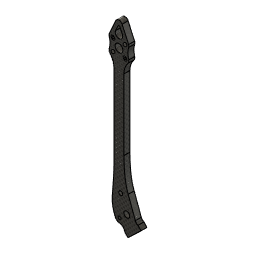
frame_assy_lab_9 (Autodesk Fusion 360 archive; units mm, degrees)
design "arm_rear_6mm"
Autodesk Fusion 360 part; units mm, degrees
(part 1 of 5)
sketch "Sketch1" plane through (0, 0, 0) normal (0, 0, 1) x (1, 0, 0)
  circle A0 centre (0, 0) radius 3.95
  line L0 (0, 0) -> (0, -178.3291)
  line L1 (-5, 0) -> (-5, -178.3291)
  line L2 (5, 0) -> (5, -178.3291)
  dimension "d1" = 7.9
  dimension "d2" = 5
  dimension "d3" = -5
  constraint coincident A0.centre L0.start
  constraint vertical L0
  measures "d1" diameter of A0
sketch "Sketch2" plane through (0, 0, 0) normal (0, 0, 1) x (1, 0, 0)
  circle A0 centre (0, 0) radius 3.95
  line L0 (0, 0) -> (-9, 0) construction
  line L1 (7.566, -7.566) -> (4.5962, -4.5962) construction
  line L2 (6.7175, 4.5962) -> (7.566, 5.4447)
  line L3 (4.5962, -6.7175) -> (5.4447, -7.566)
  line L4 (0.9091, 19.0167) -> (3.409, 13.5625)
  circle A1 centre (6.5054, -6.5054) radius 3.5
  line L5 (-4.5962, 6.7175) -> (-5.4447, 7.566)
  arc A2 (4.5962, 6.7175) -> (6.7175, 4.5962) centre (5.6569, 5.6569) ccw
  arc A3 (-7.566, -5.4447) -> (-5.4447, -7.566) centre (-6.5054, -6.5054) ccw
  arc A4 (9.1588, -8.7878) -> (5, -20) centre (22.1936, -20) ccw
  line L6 (7.566, -5.4447) -> (6.7175, -4.5962)
  arc A5 (9.8421, 5.4488) -> (9.8421, -5.4488) centre (27.0494, 0) ccw
  arc A6 (-4.5962, -6.7175) -> (-6.7175, -4.5962) centre (-5.6569, -5.6569) ccw
  circle A7 centre (0, 21) radius 3.5
  circle A8 centre (0, 12) radius 3.75
  line L7 (-5, -20) -> (5, -20) construction
  line L8 (-0.9091, 19.0167) -> (-3.409, 13.5625)
  arc A9 (5.4447, -7.566) -> (7.566, -5.4447) centre (6.5054, -6.5054) ccw
  line L9 (-6.7175, -4.5962) -> (-7.566, -5.4447)
  arc A10 (-5, -20) -> (-9.1588, -8.7878) centre (-22.1936, -20) ccw
  line L10 (5.4447, 7.566) -> (4.5962, 6.7175)
  line L11 (0, 0) -> (18.7579, 0) construction
  circle A11 centre (-6.5054, -6.5054) radius 3.5
  line L12 (-9.6985, 7.9385) -> (-3.1931, 22.4331)
  arc A12 (6.7175, -4.5962) -> (4.5962, -6.7175) centre (5.6569, -5.6569) ccw
  arc A13 (7.566, 5.4447) -> (5.4447, 7.566) centre (6.5054, 6.5054) ccw
  circle A14 centre (-6.5054, 6.5054) radius 3.5
  line L13 (0, 0) -> (13.2638, -13.2638) construction
  line L14 (0, 24.5) -> (0, 0) construction
  line L15 (9.6985, 7.9385) -> (3.1931, 22.4331)
  arc A15 (-6.7175, 4.5962) -> (-4.5962, 6.7175) centre (-5.6569, 5.6569) ccw
  line L16 (-5.4447, -7.566) -> (-4.5962, -6.7175)
  line L17 (-7.566, 5.4447) -> (-6.7175, 4.5962)
  arc A16 (-5.4447, 7.566) -> (-7.566, 5.4447) centre (-6.5054, 6.5054) ccw
  arc A17 (-9.8421, -5.4488) -> (-9.8421, 5.4488) centre (-27.0494, 0) ccw
  circle A18 centre (6.5054, 6.5054) radius 3.5
  arc A19 (0.9091, 19.0167) -> (-0.9091, 19.0167) centre (0, 18.6) ccw
  arc A20 (16.4975, -142.4127) -> (19.1132, -145.1691) centre (20.2426, -141.4781) ccw
  circle A21 centre (28.5466, -163.0999) radius 2.95 construction
  line L18 (36.8072, -178.2122) -> (44.0178, -178.0032) construction
  line L19 (-6.1772, -125.1087) -> (-6.7634, -132.2985)
  line L20 (0.7848, -157.6755) -> (0.9047, -157.0861) construction
  arc A22 (12.4548, -169.2574) -> (12.1429, -164.1911) centre (12.0783, -166.7378) ccw construction
  circle A23 centre (0.6152, -147.9032) radius 1.5
  line L21 (5.9477, -157.6628) -> (12.1429, -164.1911)
  arc A24 (5.9477, -157.6628) -> (0.9047, -157.0861) centre (3.4011, -157.594) ccw
  arc A25 (-7.3343, -135.681) -> (-6.7634, -132.2985) centre (-26.6972, -130.6734) ccw construction
  arc A26 (10.3319, -168.8201) -> (11.86, -169.3463) centre (11.6013, -167.6155) ccw construction
  arc A27 (44.0178, -178.0032) -> (46.9539, -162.6605) centre (43.7859, -170.0066) ccw construction
  arc A28 (36.8072, -178.2122) -> (33.3994, -178.6053) centre (37.3868, -198.2038) ccw construction
  arc A29 (9.2981, -122.9795) -> (-6.1772, -125.1087) centre (1.7963, -125.7587) ccw construction
  line L22 (-7.3343, -135.681) -> (-10.3423, -147.312) construction
  circle A30 centre (21.61, -170.0271) radius 1.5 construction
  line L23 (21.627, -181.0005) -> (33.3994, -178.6053) construction
  arc A31 (0.7848, -157.6755) -> (1.2303, -159.229) centre (2.4997, -158.0244) ccw construction
  line L24 (46.9539, -162.6605) -> (27.9242, -154.4539) construction
  circle A32 centre (1.7963, -125.7587) radius 2
  line L25 (10.3319, -168.8201) -> (1.2303, -159.229) construction
  line L26 (12.4548, -169.2574) -> (11.86, -169.3463) construction
  circle A33 centre (43.7859, -170.0066) radius 2 construction
  line L27 (25.3084, -151.6975) -> (19.1132, -145.1691)
  line L28 (16.4975, -142.4127) -> (9.2981, -122.9795)
  arc A34 (25.3084, -151.6975) -> (27.9242, -154.4539) centre (29.0536, -150.7628) ccw construction
  circle A35 centre (7.8959, -141.3387) radius 2.95
  circle A36 centre (0.6152, -147.9032) radius 4.5
  spline S0 degree 5 poles (0.6152, -152.4032) (0.9218, -152.4032) (1.5117, -152.4518) (2.3269, -152.6706) (3.2887, -153.2145) (4.3168, -154.1801) (5.002, -155.1015) (5.4252, -155.8554) (5.6626, -156.3853) (5.77, -156.657) knots 0 0 0 0 0 0 0.2 0.4 0.6 0.8 1 1 1 1 1 1
  line L29 (22.2108, -148.4333) -> (9.0453, -160.927)
  spline S1 degree 5 poles (-6.7634, -132.2985) (-6.8228, -133.0274) (-6.8958, -134.4803) (-6.8677, -136.6451) (-6.5849, -139.5032) (-5.9007, -143.0251) (-5.105, -145.7887) (-4.35, -147.8195) (-3.7693, -149.1519) (-3.4595, -149.8128) knots 0 0 0 0 0 0 0.2 0.4 0.6 0.8 1 1 1 1 1 1
  line L30 (0, 0) -> (0, -133.0837) construction
  line L31 (-5, 0) -> (-5, -133.0837)
  line L32 (5, 0) -> (5, -133.0837)
  spline S2 degree 5 poles (-6.1772, -125.1087) (-6.1092, -124.2742) (-5.9743, -122.6052) (-5.7752, -120.101) (-5.5198, -116.7611) (-5.2405, -112.5839) (-5.0796, -109.2394) (-5.0145, -106.7287) (-5, -105.0538) (-5, -104.2161) knots 0 0 0 0 0 0 0.2 0.4 0.6 0.8 1 1 1 1 1 1
  spline S3 degree 5 poles (9.2981, -122.9795) (8.8487, -121.7665) (8.0283, -119.3245) (7.033, -115.6132) (6.1133, -110.5828) (5.4305, -104.2105) (5.1351, -99.0813) (5.0246, -95.2302) (5, -92.6623) (5, -91.3783) knots 0 0 0 0 0 0 0.2 0.4 0.6 0.8 1 1 1 1 1 1
  point P0 (0, 24.5)
  dimension "d5" = 360
  dimension "d6" = 45
  dimension "d7" = 3
  dimension "d8" = 6.5
  dimension "d9" = 4.2
  dimension "d10" = 7
  dimension "d11" = 24.5
  dimension "d12" = 7
  dimension "d13" = 7
  dimension "d14" = 9
  dimension "d15" = 20
  dimension "d16" = 7.5
  dimension "d17" = 12
  dimension "d18" = 1
  dimension "d19" = 9
  dimension "d20" = 5
  dimension "d21" = -5
  constraint horizontal L11
  constraint coincident A0.centre L0.start
  constraint tangent L6 A12
  constraint tangent L3 A12
  constraint parallel L3 L6
  constraint tangent L3 A9
  constraint tangent L6 A9
  constraint midpoint L1.start A9
  constraint midpoint L1.end A12
  constraint coincident L1.end L13
  constraint parallel L1 L13
  constraint coincident P0 L14.start
  constraint perpendicular L11 L14
  constraint coincident P0 A7
  constraint concentric A14 A16
  constraint concentric A3 A11
  constraint perpendicular L0 L14
  constraint coincident L0.end A17
  constraint coincident A17.end A14
  constraint coincident A17.start A11
  constraint tangent A14 A17
  constraint tangent A11 A17
  constraint horizontal L7
  constraint tangent A10 A11
  constraint coincident A10.end A11
  constraint coincident A7.centre L14
  constraint coincident L12.start A14
  constraint coincident L12.end A7
  constraint tangent A7 L12
  constraint tangent L12 A14
  constraint symmetric L7.start A4.end L14
  constraint symmetric A14 L14 A18
  constraint symmetric A17.start A5.end L14
  constraint symmetric A17.end A5.start L14
  constraint symmetric A5 L14 A17
  constraint symmetric A10.end A4.start L14
  constraint symmetric A4 A10 L14
  constraint symmetric L12.start L15.start L14
  constraint symmetric L12.end L15.end L14
  constraint symmetric A1 A11 L14
  constraint coincident A8.centre L14
  constraint coincident L4.end A8
  constraint tangent L4 A8
  constraint coincident L8.end A8
  constraint tangent A8 L8
  constraint tangent L4 A19
  constraint tangent L8 A19
  constraint concentric A23 A36
  constraint coincident A36 S0.start
  constraint coincident A24 S0.end
  constraint tangent A24 S0
  constraint tangent A36 S0
  constraint midpoint L27 L29.start
  constraint midpoint L21 L29.end
  constraint coincident A36 S1.end
  constraint tangent A36 S1
  constraint perpendicular L7 L30
  constraint coincident L31 S2.end
  constraint coincident L32 S3.end
  measures "d6" angle of L11 L13
  measures "d7" diameter of A12
  measures "d8" distance of A0.centre L1.end
  measures "d9" distance of L1.start L1.end
  measures "d10" diameter of A7
  measures "d11" distance of P0 A0.centre
  measures "d12" diameter of A14
  measures "d13" diameter of A11
  measures "d14" distance of L0.end A0.centre
  measures "d15" distance of A0.centre L7
  measures "d16" diameter of A8
  measures "d17" distance of A8.centre A0.centre
  measures "d18" radius of A19
  measures "d19" diameter of A36
extrude "Extrude1" add sketch "Sketch2" along normal blind 6 contours L3 A1 A12 L32 | L3 A1 L6 A9 A12 L32 | L4 A1 A5 A7 A8 L8 A11 L12 A14 L15 A17 A18 A20 L19 L21 A24 L27 L28 A36 S0 L29 S1 L31 L32 S2 S3 | A1 A4 L32 | A18 | L4 A7 L8 A19 | A14 | A3 A6 L9 A11 L16 L31 | A10 A11 L31 | A6 A11 L16 L31 | A36 picked at (0.167, 22.8547)

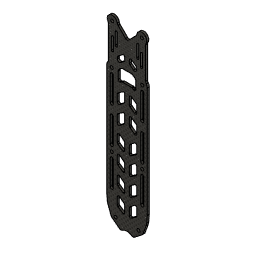
design "top_plate_2mm"
Autodesk Fusion 360 part; units mm, degrees
sketch "Sketch1" plane through (0, 0, 0) normal (0, 0, 1) x (1, 0, 0)
  line L0 (6.189, -57.15) -> (-6.189, -57.15) construction
  arc A0 (33.9547, -44.6156) -> (27.7114, -50.1961) centre (40.4322, -58.1449) ccw construction
  line L1 (-7.8851, -56.2098) -> (-15.1961, -44.5098) construction
  line L2 (15.1961, -44.5098) -> (7.8851, -56.2098) construction
  line L3 (5.15, -89.2) -> (-5.15, -89.2) construction
  arc A1 (6.189, -57.15) -> (7.8851, -56.2098) centre (6.189, -55.15) ccw construction
  arc A2 (-7.8851, -56.2098) -> (-6.189, -57.15) centre (-6.189, -55.15) ccw construction
  arc A3 (-27.7114, -50.1961) -> (-33.9547, -44.6156) centre (-40.4322, -58.1449) ccw construction
  arc A4 (21.55, -94.9296) -> (23.2215, -100.7587) centre (32.55, -94.9296) ccw construction
  line L4 (-5.15, -68.9) -> (5.15, -68.9) construction
  line L5 (21.55, -94.9296) -> (21.55, -63.2107) construction
  line L6 (-7.65, -86.7) -> (-7.65, -71.4) construction
  line L7 (-21.55, -63.2107) -> (-21.55, -94.9296) construction
  line L8 (7.65, -71.4) -> (7.65, -86.7) construction
  line L9 (-27.7114, -50.1961) -> (-23.2215, -57.3816) construction
  arc A5 (-5.15, -68.9) -> (-7.65, -71.4) centre (-5.15, -71.4) ccw construction
  circle A6 centre (15.25, -63.8) radius 2.95 construction
  arc A7 (23.2215, -57.3816) -> (21.55, -63.2107) centre (32.55, -63.2107) ccw construction
  arc A8 (5.15, -89.2) -> (7.65, -86.7) centre (5.15, -86.7) ccw construction
  arc A9 (7.65, -71.4) -> (5.15, -68.9) centre (5.15, -71.4) ccw construction
  arc A10 (-14.75, 10.1) -> (-19, 2.4661) centre (-14.75, 5.1) ccw construction
  arc A11 (-6.0958, -43.2074) -> (-10.3384, -41.45) centre (-10.3384, -47.45) ccw construction
  line L10 (-2.35, -6.7029) -> (-2.35, -10.5206) construction
  arc A12 (8.0447, -101.6962) -> (6.6112, -100.95) centre (6.6112, -102.7) ccw construction
  arc A13 (-5.4482, 6.3017) -> (-5.6227, 4.1031) centre (-4.9486, 5.1558) ccw construction
  line L11 (10.3384, -41.45) -> (13.5, -41.45) construction
  arc A14 (-15.55, -20.5) -> (-13.55, -20.5) centre (-14.55, -20.5) ccw construction
  line L12 (-15.55, -20.5) -> (-15.55, -8.5) construction
  line L13 (-18.55, 0.8857) -> (-18.55, -26.4) construction
  arc A15 (6.43, -26.8244) -> (9.65, -25.2396) centre (7.65, -25.2396) ccw construction
  arc A16 (-4.5, -123.6) -> (-8.3, -123.6) centre (-6.4, -126.96) ccw construction
  line L14 (15.55, -8.5) -> (15.55, -20.5) construction
  arc A17 (-30.5, -29.4) -> (-33.9547, -44.6156) centre (-30.5, -37.4) ccw construction
  line L15 (3.3637, -4.8501) -> (5.7029, -3.3523) construction
  line L16 (-13.7095, 10.1) -> (-14.75, 10.1) construction
  line L17 (8.0447, -101.6962) -> (8.3897, -102.1889) construction
  line L18 (-13.5, -41.45) -> (-10.3384, -41.45) construction
  line L19 (30.5, -29.4) -> (21.55, -29.4) construction
  arc A18 (-11.75, -14.5) -> (-9.75, -14.5) centre (-10.75, -14.5) ccw construction
  line L20 (9.65, -23.8089) -> (9.65, -25.2396) construction
  line L21 (-13.55, -8.5) -> (-13.55, -20.5) construction
  arc A19 (15.1961, -44.5098) -> (13.5, -41.45) centre (13.5, -43.45) ccw construction
  line L22 (13.55, -20.5) -> (13.55, -8.5) construction
  line L23 (-7.55, -11.0338) -> (-7.55, -4.3629) construction
  line L24 (18.55, -26.4) -> (18.55, 0.8857) construction
  arc A20 (-9.65, -25.2396) -> (-6.43, -26.8244) centre (-7.65, -25.2396) ccw construction
  line L25 (-5.7029, -3.3523) -> (-3.3637, -4.8501) construction
  arc A21 (-9.75, -2.5) -> (-11.75, -2.5) centre (-10.75, -2.5) ccw construction
  circle A22 centre (-15.25, -35.5) radius 1.5
  line L26 (-8.8217, -22.188) -> (-4.253, -18.8853) construction
  circle A23 centre (15.25, -108.3) radius 1.5
  line L27 (-31.6483, -113.6894) -> (-36.4601, -119.0636) construction
  line L28 (4.253, -18.8853) -> (8.8217, -22.188) construction
  line L29 (29.5877, -110.9469) -> (23.2215, -100.7587) construction
  line L30 (9.75, -14.5) -> (9.75, -2.5) construction
  circle A24 centre (15, -118.1) radius 2.95 construction
  line L31 (6.43, -26.8244) -> (2.818, -24.044) construction
  arc A25 (-8.3897, -102.1889) -> (-4.5, -105.45) centre (-6.3028, -103.6501) ccw construction
  arc A26 (13.55, -20.5) -> (15.55, -20.5) centre (14.55, -20.5) ccw construction
  line L32 (-21.55, -29.4) -> (-30.5, -29.4) construction
  line L33 (-27.3521, -131.7546) -> (-8.3, -123.6) construction
  line L34 (2.35, -23.0931) -> (2.35, -19.8578) construction
  line L35 (-6.0958, -43.2074) -> (-4.8532, -44.45) construction
  line L36 (-9.65, -25.2396) -> (-9.65, -23.8089) construction
  line L37 (-2.35, -19.8578) -> (-2.35, -23.0931) construction
  line L38 (-11.75, -14.5) -> (-11.75, -2.5) construction
  line L39 (-1.3481, 1.3661) -> (-5.6227, 4.1031) construction
  arc A27 (-7.55, -11.0338) -> (-4.1622, -12.8855) centre (-5.35, -11.0338) ccw construction
  line L40 (-8.3897, -102.1889) -> (-8.0447, -101.6962) construction
  arc A28 (18.55, -26.4) -> (21.55, -29.4) centre (21.55, -26.4) ccw construction
  circle A29 centre (-30.5, -37.4) radius 2 construction
  circle A30 centre (14.75, 5.1) radius 1.5
  circle A31 centre (-14.75, 5.1) radius 1.5
  arc A32 (-13.5, -41.45) -> (-15.1961, -44.5098) centre (-13.5, -43.45) ccw construction
  arc A33 (33.9547, -44.6156) -> (30.5, -29.4) centre (30.5, -37.4) ccw construction
  arc A34 (-5.7029, -3.3523) -> (-7.55, -4.3629) centre (-6.35, -4.3629) ccw construction
  line L41 (4.1622, -12.8855) -> (3.3622, -12.3724) construction
  arc A35 (-2.818, -24.044) -> (-2.35, -23.0931) centre (-3.55, -23.0931) ccw construction
  arc A36 (-3.3622, -12.3724) -> (-2.35, -10.5206) centre (-4.55, -10.5206) ccw construction
  arc A37 (0.3197, 8.5373) -> (-0.3197, 8.5373) centre (0, 7.804) ccw construction
  line L42 (-9.75, -2.5) -> (-9.75, -14.5) construction
  arc A38 (2.35, -10.5206) -> (3.3622, -12.3724) centre (4.55, -10.5206) ccw construction
  line L43 (0.3197, 8.5373) -> (5.4482, 6.3017) construction
  arc A39 (15.55, -8.5) -> (13.55, -8.5) centre (14.55, -8.5) ccw construction
  line L44 (-2.818, -24.044) -> (-6.43, -26.8244) construction
  arc A40 (19, 2.4661) -> (14.75, 10.1) centre (14.75, 5.1) ccw construction
  arc A41 (-8.8217, -22.188) -> (-9.65, -23.8089) centre (-7.65, -23.8089) ccw construction
  arc A42 (-18.55, 0.8857) -> (-19, 2.4661) centre (-21.55, 0.8857) ccw construction
  line L45 (-2.7973, 14.2208) -> (-10.9121, 10.6832) construction
  line L46 (7.55, -4.3629) -> (7.55, -11.0338) construction
  arc A43 (3.3637, -4.8501) -> (2.35, -6.7029) centre (4.55, -6.7029) ccw construction
  arc A44 (11.75, -2.5) -> (9.75, -2.5) centre (10.75, -2.5) ccw construction
  line L47 (11.75, -2.5) -> (11.75, -14.5) construction
  arc A45 (-13.55, -8.5) -> (-15.55, -8.5) centre (-14.55, -8.5) ccw construction
  arc A46 (10.9121, 10.6832) -> (13.7095, 10.1) centre (13.7095, 17.1) ccw construction
  arc A47 (5.6227, 4.1031) -> (5.4482, 6.3017) centre (4.9486, 5.1558) ccw construction
  line L48 (14.75, 10.1) -> (13.7095, 10.1) construction
  line L49 (2.35, -10.5206) -> (2.35, -6.7029) construction
  line L50 (5.6227, 4.1031) -> (1.3481, 1.3661) construction
  arc A48 (9.75, -14.5) -> (11.75, -14.5) centre (10.75, -14.5) ccw construction
  arc A49 (4.1622, -12.8855) -> (7.55, -11.0338) centre (5.35, -11.0338) ccw construction
  arc A50 (7.55, -4.3629) -> (5.7029, -3.3523) centre (6.35, -4.3629) ccw construction
  arc A51 (19, 2.4661) -> (18.55, 0.8857) centre (21.55, 0.8857) ccw construction
  line L51 (-3.3622, -12.3724) -> (-4.1622, -12.8855) construction
  arc A52 (-2.35, -19.8578) -> (-4.253, -18.8853) centre (-3.55, -19.8578) ccw construction
  arc A53 (-2.35, -6.7029) -> (-3.3637, -4.8501) centre (-4.55, -6.7029) ccw construction
  arc A54 (-21.55, -29.4) -> (-18.55, -26.4) centre (-21.55, -26.4) ccw construction
  line L52 (10.9121, 10.6832) -> (2.7973, 14.2208) construction
  arc A55 (-13.7095, 10.1) -> (-10.9121, 10.6832) centre (-13.7095, 17.1) ccw construction
  circle A56 centre (-15.25, -63.8) radius 2.95 construction
  line L53 (4.8532, -44.45) -> (6.0958, -43.2074) construction
  arc A57 (29.5877, -110.9469) -> (31.6483, -113.6894) centre (46.5487, -100.3485) ccw construction
  arc A58 (4.253, -18.8853) -> (2.35, -19.8578) centre (3.55, -19.8578) ccw construction
  arc A59 (10.3384, -41.45) -> (6.0958, -43.2074) centre (10.3384, -47.45) ccw construction
  arc A60 (27.3521, -131.7546) -> (36.4601, -119.0636) centre (30.5, -124.4) ccw construction
  arc A61 (-36.4601, -119.0636) -> (-27.3521, -131.7546) centre (-30.5, -124.4) ccw construction
  circle A62 centre (-15.25, -94.3) radius 2.95 construction
  line L54 (36.4601, -119.0636) -> (31.6483, -113.6894) construction
  arc A63 (4.5, -105.45) -> (8.3897, -102.1889) centre (6.3028, -103.6501) ccw construction
  line L55 (-23.2215, -100.7587) -> (-29.5877, -110.9469) construction
  line L56 (8.3, -123.6) -> (27.3521, -131.7546) construction
  line L57 (-5.4482, 6.3017) -> (-0.3197, 8.5373) construction
  line L58 (4.5, -105.45) -> (-4.5, -105.45) construction
  arc A64 (2.35, -23.0931) -> (2.818, -24.044) centre (3.55, -23.0931) ccw construction
  arc A65 (-1.3481, 1.3661) -> (1.3481, 1.3661) centre (0, 3.4715) ccw construction
  arc A66 (-23.2215, -100.7587) -> (-21.55, -94.9296) centre (-32.55, -94.9296) ccw construction
  line L59 (-6.6112, -100.95) -> (6.6112, -100.95) construction
  circle A67 centre (-30.5, -124.4) radius 2 construction
  line L60 (-4.5, -123.6) -> (4.5, -123.6) construction
  arc A68 (9.65, -23.8089) -> (8.8217, -22.188) centre (7.65, -23.8089) ccw construction
  arc A69 (2.7973, 14.2208) -> (-2.7973, 14.2208) centre (0, 7.804) ccw construction
  circle A70 centre (30.5, -37.4) radius 2 construction
  circle A71 centre (-15.25, -108.3) radius 1.5
  circle A72 centre (-15, -118.1) radius 2.95 construction
  circle A73 centre (30.5, -124.4) radius 2 construction
  arc A74 (-6.6112, -100.95) -> (-8.0447, -101.6962) centre (-6.6112, -102.7) ccw construction
  circle A75 centre (15.25, -94.3) radius 2.95 construction
  circle A76 centre (15.25, -35.5) radius 1.5
  arc A77 (8.3, -123.6) -> (4.5, -123.6) centre (6.4, -126.96) ccw construction
  line L61 (-4.8532, -44.45) -> (4.8532, -44.45) construction
  arc A78 (-31.6483, -113.6894) -> (-29.5877, -110.9469) centre (-46.5487, -100.3485) ccw construction
  line L62 (23.2215, -57.3816) -> (27.7114, -50.1961) construction
  arc A79 (-21.55, -63.2107) -> (-23.2215, -57.3816) centre (-32.55, -63.2107) ccw construction
  arc A80 (-7.65, -86.7) -> (-5.15, -89.2) centre (-5.15, -86.7) ccw construction
  line L63 (21.55, -94.9296) -> (21.55, -63.2107) construction
  line L64 (5.45, -68.479) -> (5.45, -89.621) construction
  circle A81 centre (10, -69.05) radius 1.5 construction
  circle A82 centre (10, -89.05) radius 1.5 construction
  line L65 (-21.55, -63.2107) -> (-21.55, -94.9296) construction
  circle A83 centre (-10, -89.05) radius 1.5 construction
  arc A84 (5.2981, -91.3575) -> (5.45, -89.621) centre (-4.55, -89.621) ccw construction
  arc A85 (5.45, -68.479) -> (5.2981, -66.7425) centre (-4.55, -68.479) ccw construction
  circle A86 centre (30.5, -37.4) radius 3.375 construction
  arc A87 (10.3384, -41.45) -> (6.0958, -43.2074) centre (10.3384, -47.45) ccw construction
  arc A88 (33.9547, -44.6156) -> (27.7114, -50.1961) centre (40.4322, -58.1449) ccw construction
  arc A89 (3.2687, -128.2504) -> (2.5, -129.8265) centre (4.5, -129.8265) ccw construction
  line L66 (5.0629, -146.1617) -> (5.25, -146.1617) construction
  arc A90 (9.1581, -153.5522) -> (8.9013, -150.8916) centre (8.3519, -152.2873) ccw construction
  line L67 (29.5877, -110.9469) -> (23.2215, -100.7587) construction
  arc A91 (22.987, -129.8863) -> (20.2, -131.7249) centre (22.2, -131.7249) ccw construction
  circle A92 centre (-10, -148.1) radius 1 construction
  arc A93 (7.0571, -163.8147) -> (3.1079, -160.45) centre (3.1079, -164.45) ccw construction
  arc A94 (-8.9013, -150.8916) -> (-7, -148.1) centre (-10, -148.1) ccw construction
  arc A95 (9.532, -132.1468) -> (8.688, -130.7979) centre (8.032, -132.1468) ccw construction
  arc A96 (7.3512, -129.5084) -> (8.688, -130.7979) centre (10, -128.1) ccw construction
  line L68 (2.5, -137.5767) -> (2.5, -129.8265) construction
  line L69 (-3.1079, -160.45) -> (3.1079, -160.45) construction
  line L70 (-5.25, -146.1617) -> (-5.0629, -146.1617) construction
  arc A97 (-9.532, -134.0551) -> (-8.8457, -135.3152) centre (-8.032, -134.0551) ccw construction
  line L71 (15.7286, -164.6391) -> (19.1143, -155.3371) construction
  line L72 (-4.1394, -146.4797) -> (-3.0765, -147.3101) construction
  circle A98 centre (-11.5, -163.1) radius 1.5
  arc A99 (29.5877, -110.9469) -> (31.6483, -113.6894) centre (46.5487, -100.3485) ccw construction
  circle A100 centre (-10, -128.1) radius 1 construction
  arc A101 (-15.7286, -164.6391) -> (-7.0571, -163.8147) centre (-11.5, -163.1) ccw construction
  circle A102 centre (11.5, -163.1) radius 1.5
  line L73 (5.2981, -91.3575) -> (4.4577, -96.1236) construction
  arc A103 (-4.0375, -156.816) -> (-2.5, -155.9727) centre (-3.5, -155.9727) ccw construction
  line L74 (7, -147.9117) -> (7, -148.1) construction
  arc A104 (-8.688, -130.7979) -> (-9.532, -132.1468) centre (-8.032, -132.1468) ccw construction
  line L75 (22.987, -129.8863) -> (27.3521, -131.7546) construction
  arc A105 (-2.5, -148.4921) -> (-3.0765, -147.3101) centre (-4, -148.4921) ccw construction
  arc A106 (2.5, -137.5767) -> (4.0425, -138.4168) centre (3.5, -137.5767) ccw construction
  arc A107 (-3.1079, -160.45) -> (-7.0571, -163.8147) centre (-3.1079, -164.45) ccw construction
  circle A108 centre (10, -128.1) radius 1 construction
  arc A109 (19.1143, -155.3371) -> (19.6835, -152.7386) centre (9.7173, -151.9169) ccw construction
  arc A110 (-4.1394, -146.4797) -> (-5.0629, -146.1617) centre (-5.0629, -147.6617) ccw construction
  arc A111 (7, -148.1) -> (8.9013, -150.8916) centre (10, -148.1) ccw construction
  line L76 (19.6835, -152.7386) -> (20.1662, -146.8849) construction
  line L77 (-23.2215, -100.7587) -> (-29.5877, -110.9469) construction
  arc A112 (3.4729, -96.95) -> (4.4577, -96.1236) centre (3.4729, -95.95) ccw construction
  arc A113 (5.0629, -146.1617) -> (4.1394, -146.4797) centre (5.0629, -147.6617) ccw construction
  line L78 (3.4729, -96.95) -> (-3.4729, -96.95) construction
  line L79 (9.1581, -153.5522) -> (4.0375, -156.816) construction
  arc A114 (2.5, -155.9727) -> (4.0375, -156.816) centre (3.5, -155.9727) ccw construction
  line L80 (3.0765, -147.3101) -> (4.1394, -146.4797) construction
  circle A115 centre (15, -148.1) radius 1.5 construction
  line L81 (6.7994, -128.4707) -> (7.3512, -129.5084) construction
  line L82 (9.532, -132.1468) -> (9.532, -134.0551) construction
  arc A116 (7, -147.9117) -> (5.25, -146.1617) centre (5.25, -147.9117) ccw construction
  line L83 (8.8457, -135.3152) -> (4.0425, -138.4168) construction
  circle A117 centre (15.25, -94.3) radius 1.5 construction
  arc A118 (7.0571, -163.8147) -> (15.7286, -164.6391) centre (11.5, -163.1) ccw construction
  line L84 (-7, -148.1) -> (-7, -147.9117) construction
  arc A119 (3.0765, -147.3101) -> (2.5, -148.4921) centre (4, -148.4921) ccw construction
  arc A120 (21.55, -94.9296) -> (23.2215, -100.7587) centre (32.55, -94.9296) ccw construction
  line L85 (4.5, -105.45) -> (-4.5, -105.45) construction
  line L86 (2.5, -155.9727) -> (2.5, -148.4921) construction
  arc A121 (-8.9013, -150.8916) -> (-9.1581, -153.5522) centre (-8.3519, -152.2873) ccw construction
  arc A122 (8.8457, -135.3152) -> (9.532, -134.0551) centre (8.032, -134.0551) ccw construction
  circle A123 centre (30.5, -124.4) radius 3.375 construction
  line L87 (-20.2, -131.7249) -> (-20.2, -146.0632) construction
  line L88 (36.4601, -119.0636) -> (31.6483, -113.6894) construction
  line L89 (-6.6112, -100.95) -> (6.6112, -100.95) construction
  circle A124 centre (15.25, -108.3) radius 1.5 construction
  arc A125 (-3.4729, -61.15) -> (-4.4577, -61.9764) centre (-3.4729, -62.15) ccw construction
  line L90 (8.0447, -101.6962) -> (8.3897, -102.1889) construction
  line L91 (3.2687, -128.2504) -> (3.8022, -127.8336) construction
  circle A126 centre (15, -118.1) radius 1.5 construction
  arc A127 (6.7994, -128.4707) -> (3.8022, -127.8336) centre (5.0335, -129.4096) ccw construction
  line L92 (-3.4729, -61.15) -> (3.4729, -61.15) construction
  line L93 (-4.8532, -44.45) -> (4.8532, -44.45) construction
  arc A128 (4.5, -105.45) -> (8.3897, -102.1889) centre (6.3028, -103.6501) ccw construction
  arc A129 (8.0447, -101.6962) -> (6.6112, -100.95) centre (6.6112, -102.7) ccw construction
  line L94 (6.189, -55.85) -> (-6.189, -55.85) construction
  arc A130 (-21.55, -63.2107) -> (-23.2215, -57.3816) centre (-32.55, -63.2107) ccw construction
  arc A131 (-30.5, -29.4) -> (-33.9547, -44.6156) centre (-30.5, -37.4) ccw construction
  line L95 (20.2, -146.0632) -> (20.2, -131.7249) construction
  arc A132 (27.3521, -131.7546) -> (36.4601, -119.0636) centre (30.5, -124.4) ccw construction
  arc A133 (-36.4601, -119.0636) -> (-27.3521, -131.7546) centre (-30.5, -124.4) ccw construction
  line L96 (-7.3512, -129.5084) -> (-6.7994, -128.4707) construction
  line L97 (-27.3521, -131.7546) -> (-22.987, -129.8863) construction
  circle A134 centre (-15, -118.1) radius 1.5 construction
  arc A135 (20.1662, -146.8849) -> (20.2, -146.0632) centre (10.2, -146.0632) ccw construction
  arc A136 (-19.6835, -152.7386) -> (-19.1143, -155.3371) centre (-9.7173, -151.9169) ccw construction
  circle A137 centre (-15, -148.1) radius 1.5 construction
  arc A138 (-20.2, -146.0632) -> (-20.1662, -146.8849) centre (-10.2, -146.0632) ccw construction
  circle A139 centre (-15.25, -108.3) radius 1.5 construction
  arc A140 (-3.8022, -127.8336) -> (-6.7994, -128.4707) centre (-5.0335, -129.4096) ccw construction
  circle A141 centre (-15.25, -94.3) radius 1.5 construction
  line L98 (-9.532, -134.0551) -> (-9.532, -132.1468) construction
  line L99 (-4.4577, -96.1236) -> (-5.2981, -91.3575) construction
  arc A142 (-20.2, -131.7249) -> (-22.987, -129.8863) centre (-22.2, -131.7249) ccw construction
  arc A143 (-23.2215, -100.7587) -> (-21.55, -94.9296) centre (-32.55, -94.9296) ccw construction
  circle A144 centre (10, -148.1) radius 1 construction
  line L100 (-20.1662, -146.8849) -> (-19.6835, -152.7386) construction
  arc A145 (-31.6483, -113.6894) -> (-29.5877, -110.9469) centre (-46.5487, -100.3485) ccw construction
  circle A146 centre (-30.5, -124.4) radius 3.375 construction
  line L101 (-19.1143, -155.3371) -> (-15.7286, -164.6391) construction
  line L102 (-8.3897, -102.1889) -> (-8.0447, -101.6962) construction
  line L103 (-4.0425, -138.4168) -> (-8.8457, -135.3152) construction
  arc A147 (-6.6112, -100.95) -> (-8.0447, -101.6962) centre (-6.6112, -102.7) ccw construction
  line L104 (-2.5, -148.4921) -> (-2.5, -155.9727) construction
  arc A148 (-4.0425, -138.4168) -> (-2.5, -137.5767) centre (-3.5, -137.5767) ccw construction
  line L105 (-31.6483, -113.6894) -> (-36.4601, -119.0636) construction
  arc A149 (-8.3897, -102.1889) -> (-4.5, -105.45) centre (-6.3028, -103.6501) ccw construction
  arc A150 (-8.688, -130.7979) -> (-7.3512, -129.5084) centre (-10, -128.1) ccw construction
  line L106 (-3.8022, -127.8336) -> (-3.2687, -128.2504) construction
  arc A151 (-4.4577, -96.1236) -> (-3.4729, -96.95) centre (-3.4729, -95.95) ccw construction
  line L107 (-4.0375, -156.816) -> (-9.1581, -153.5522) construction
  arc A152 (-5.25, -146.1617) -> (-7, -147.9117) centre (-5.25, -147.9117) ccw construction
  line L108 (-2.5, -129.8265) -> (-2.5, -137.5767) construction
  arc A153 (-2.5, -129.8265) -> (-3.2687, -128.2504) centre (-4.5, -129.8265) ccw construction
  line L109 (-27.7114, -50.1961) -> (-23.2215, -57.3816) construction
  arc A154 (-6.0958, -43.2074) -> (-10.3384, -41.45) centre (-10.3384, -47.45) ccw construction
  line L110 (-9.313, -29.4) -> (-30.5, -29.4) construction
  arc A155 (-9.313, -29.4) -> (-5, -26.45) centre (-9.313, -24.7722) ccw construction
  arc A156 (-13.5, -41.45) -> (-15.1961, -44.5098) centre (-13.5, -43.45) ccw construction
  line L111 (-9.0119, -54.4991) -> (-15.1961, -44.5098) construction
  line L112 (5, -26.45) -> (-5, -26.45) construction
  circle A157 centre (-30.5, -37.4) radius 3.375 construction
  arc A158 (-27.7114, -50.1961) -> (-33.9547, -44.6156) centre (-40.4322, -58.1449) ccw construction
  circle A159 centre (-10, -69.05) radius 1.5 construction
  spline S0 degree 5 poles (-6.189, -55.85) (-6.3253, -55.85) (-6.5947, -55.8392) (-6.9894, -55.7905) (-7.4965, -55.6656) (-8.0875, -55.414) (-8.5077, -55.1235) (-8.7794, -54.8402) (-8.9382, -54.6183) (-9.0119, -54.4991) knots -1 -1 -1 -1 -1 -1 -0.8 -0.6 -0.4 -0.2 0 0 0 0 0 0 construction
  circle A160 centre (-15.25, -35.5) radius 1.5 construction
  line L113 (-6.0958, -43.2074) -> (-4.8532, -44.45) construction
  line L114 (-13.5, -41.45) -> (-10.3384, -41.45) construction
  line L115 (4.4577, -61.9764) -> (5.2981, -66.7425) construction
  circle A161 centre (15.25, -63.8) radius 1.5 construction
  line L116 (15.1961, -44.5098) -> (9.0119, -54.4991) construction
  circle A162 centre (15.25, -35.5) radius 1.5 construction
  arc A163 (5, -26.45) -> (9.313, -29.4) centre (9.313, -24.7722) ccw construction
  line L117 (10.3384, -41.45) -> (13.5, -41.45) construction
  line L118 (30.5, -29.4) -> (9.313, -29.4) construction
  arc A164 (33.9547, -44.6156) -> (30.5, -29.4) centre (30.5, -37.4) ccw construction
  line L119 (4.8532, -44.45) -> (6.0958, -43.2074) construction
  spline S1 degree 5 poles (9.0119, -54.4991) (8.9382, -54.6183) (8.7794, -54.8402) (8.5077, -55.1235) (8.0875, -55.414) (7.4965, -55.6656) (6.9894, -55.7905) (6.5947, -55.8392) (6.3253, -55.85) (6.189, -55.85) knots 0 0 0 0 0 0 0.2 0.4 0.6 0.8 1 1 1 1 1 1 construction
  line L120 (23.2215, -57.3816) -> (27.7114, -50.1961) construction
  arc A165 (15.1961, -44.5098) -> (13.5, -41.45) centre (13.5, -43.45) ccw construction
  circle A166 centre (-15.25, -63.8) radius 1.5 construction
  line L121 (-5.2981, -66.7425) -> (-4.4577, -61.9764) construction
  arc A167 (23.2215, -57.3816) -> (21.55, -63.2107) centre (32.55, -63.2107) ccw construction
  arc A168 (-5.2981, -66.7425) -> (-5.45, -68.479) centre (4.55, -68.479) ccw construction
  arc A169 (4.4577, -61.9764) -> (3.4729, -61.15) centre (3.4729, -62.15) ccw construction
  line L122 (-5.45, -89.621) -> (-5.45, -68.479) construction
  arc A170 (-5.45, -89.621) -> (-5.2981, -91.3575) centre (4.55, -89.621) ccw construction
  point P0 (0, -44.45)
sketch "Sketch2" plane through (0, 0, 0) normal (0, 0, 1) x (1, 0, 0)
  circle A0 centre (14.75, 5.1) radius 1.5
  circle A1 centre (-14.75, 5.1) radius 1.5
  arc A2 (-14.75, 10.1) -> (-19, 2.4661) centre (-14.75, 5.1) ccw construction
  arc A3 (-18.55, 0.8857) -> (-19, 2.4661) centre (-21.55, 0.8857) ccw
  line L0 (-18.55, 0.8857) -> (-18.55, -26.4)
  line L1 (18.55, -26.4) -> (18.55, 0.8857)
  arc A4 (19, 2.4661) -> (18.55, 0.8857) centre (21.55, 0.8857) ccw
  arc A5 (19, 2.4661) -> (14.75, 10.1) centre (14.75, 5.1) ccw construction
  arc A6 (11.75, -2.5) -> (9.75, -2.5) centre (10.75, -2.5) ccw
  line L2 (9.75, -14.5) -> (9.75, -2.5)
  line L3 (11.75, -2.5) -> (11.75, -14.5)
  arc A7 (9.75, -14.5) -> (11.75, -14.5) centre (10.75, -14.5) ccw
  line L4 (13.55, -20.5) -> (13.55, -8.5)
  arc A8 (15.55, -8.5) -> (13.55, -8.5) centre (14.55, -8.5) ccw
  line L5 (15.55, -8.5) -> (15.55, -20.5)
  arc A9 (13.55, -20.5) -> (15.55, -20.5) centre (14.55, -20.5) ccw
  arc A10 (-13.55, -8.5) -> (-15.55, -8.5) centre (-14.55, -8.5) ccw
  line L6 (-15.55, -20.5) -> (-15.55, -8.5)
  line L7 (-13.55, -8.5) -> (-13.55, -20.5)
  arc A11 (-15.55, -20.5) -> (-13.55, -20.5) centre (-14.55, -20.5) ccw
  arc A12 (-11.75, -14.5) -> (-9.75, -14.5) centre (-10.75, -14.5) ccw
  line L8 (-9.75, -2.5) -> (-9.75, -14.5)
  line L9 (-11.75, -14.5) -> (-11.75, -2.5)
  arc A13 (-9.75, -2.5) -> (-11.75, -2.5) centre (-10.75, -2.5) ccw
  line L10 (4.253, -18.8853) -> (8.8217, -22.188)
  arc A14 (4.253, -18.8853) -> (2.35, -19.8578) centre (3.55, -19.8578) ccw
  line L11 (2.35, -23.0931) -> (2.35, -19.8578)
  line L12 (6.43, -26.8244) -> (2.818, -24.044)
  arc A15 (6.43, -26.8244) -> (9.65, -25.2396) centre (7.65, -25.2396) ccw
  arc A16 (2.35, -23.0931) -> (2.818, -24.044) centre (3.55, -23.0931) ccw
  arc A17 (9.65, -23.8089) -> (8.8217, -22.188) centre (7.65, -23.8089) ccw
  line L13 (9.65, -23.8089) -> (9.65, -25.2396)
  line L14 (-2.35, -19.8578) -> (-2.35, -23.0931)
  arc A18 (-2.35, -19.8578) -> (-4.253, -18.8853) centre (-3.55, -19.8578) ccw
  line L15 (-8.8217, -22.188) -> (-4.253, -18.8853)
  arc A19 (-8.8217, -22.188) -> (-9.65, -23.8089) centre (-7.65, -23.8089) ccw
  line L16 (-9.65, -25.2396) -> (-9.65, -23.8089)
  arc A20 (-9.65, -25.2396) -> (-6.43, -26.8244) centre (-7.65, -25.2396) ccw
  line L17 (-2.818, -24.044) -> (-6.43, -26.8244)
  arc A21 (-2.818, -24.044) -> (-2.35, -23.0931) centre (-3.55, -23.0931) ccw
  circle A22 centre (15.25, -35.5) radius 1.5
  circle A23 centre (-15.25, -35.5) radius 1.5
  circle A24 centre (-15.25, -108.3) radius 1.5
  circle A25 centre (15.25, -108.3) radius 1.5
  circle A26 centre (11.5, -163.1) radius 1.5
  circle A27 centre (-11.5, -163.1) radius 1.5
  line L18 (0, -4.9) -> (0, 10.1) construction
  line L19 (-14.75, 10.1) -> (0, 10.1) construction
  circle A28 centre (-14.75, 5.1) radius 5
  circle A29 centre (14.75, 5.1) radius 5
  line L20 (0, -4.9) -> (-9.756, 4.856)
  line L21 (0, -4.9) -> (13.797, -4.9) construction
  line L22 (0, -4.9) -> (9.756, 4.856)
  circle A30 centre (15.25, -35.5) radius 5
  circle A31 centre (-15.25, -35.5) radius 5
  line L23 (18.55, -26.4) -> (18.55, -31.7437)
  line L24 (20.25, -35.5) -> (20.25, -145.8683)
  line L25 (-18.55, -26.4) -> (-18.55, -31.7437)
  line L26 (-20.25, -35.5) -> (-20.25, -145.8683)
  line L27 (19.6835, -152.7386) -> (20.1662, -146.8849)
  arc A32 (19.1143, -155.3371) -> (19.6835, -152.7386) centre (9.7173, -151.9169) ccw
  line L28 (15.7286, -164.6391) -> (19.1143, -155.3371)
  line L29 (20.1662, -146.8849) -> (20.25, -145.8683)
  line L30 (-20.25, -145.8683) -> (20.25, -145.8683) construction
  line L31 (0, 0) -> (0, -234.4396) construction
  line L32 (15.7286, -164.6391) -> (6, -172.1)
  line L33 (6, -172.1) -> (-6, -172.1) construction
  line L34 (0, -172.1) -> (0, -169.6) construction
  circle A33 centre (0, -178.05) radius 8.45
  line L35 (-20.1662, -146.8849) -> (-20.25, -145.8683)
  line L36 (-19.6835, -152.7386) -> (-20.1662, -146.8849)
  arc A34 (-19.6835, -152.7386) -> (-19.1143, -155.3371) centre (-9.7173, -151.9169) ccw
  line L37 (-15.7286, -164.6391) -> (-19.1143, -155.3371)
  line L38 (-15.7286, -164.6391) -> (-6, -172.1)
  point P0 (6, -172.1)
  dimension "d1" = 15
  dimension "d2" = 135
  dimension "d3" = 10
  dimension "d4" = 10
  dimension "d7" = 9
  dimension "d8" = 6
  dimension "d9" = 12
  dimension "d10" = 2.5
  constraint coincident A2.start L19.start
  constraint tangent A2 L19
  constraint concentric A2 A28
  constraint coincident A2.end A28
  constraint concentric A5 A29
  constraint coincident A4.start A29
  constraint horizontal L21
  constraint coincident A28 L20.end
  constraint coincident A29 L22.end
  constraint perpendicular L20 L22
  constraint concentric A22 A30
  constraint concentric A23 A31
  constraint coincident L1.start L23.start
  constraint coincident A30 L23.end
  constraint parallel L1 L23
  constraint coincident A30 L24.start
  constraint tangent A30 L24
  constraint parallel L23 L24
  constraint coincident L0.end L25.start
  constraint coincident A31 L25.end
  constraint parallel L0 L25
  constraint coincident A31 L26.start
  constraint vertical L26
  constraint tangent A31 L26
  constraint coincident L27.end L29.start
  constraint collinear L27 L29
  constraint horizontal L30
  constraint coincident L31.start origin
  constraint perpendicular L21 L31
  constraint coincident L28.start L32.start
  constraint coincident P0 L32.end
  constraint horizontal L33
  constraint midpoint L33 L34.start
  constraint perpendicular L33 L34
  constraint coincident L33.end A33
  constraint coincident P0 A33
  constraint coincident L34.end A33
  constraint symmetric L24.end L31 L26.end
  constraint symmetric L27.start L31 L36.start
  constraint symmetric L27.end L31 L35.start
  constraint symmetric A32.start L31 A34.end
  constraint symmetric A32 L31 A34
  constraint symmetric L28.start L31 L37.start
  constraint symmetric L31 L28.start L37.start
  constraint symmetric L31 P0 L33.end
  measures "d1" distance of L18.start L18.end
  measures "d2" angle of L20 L21
  measures "d3" diameter of A30
  measures "d4" diameter of A31
  measures "d7" vertical distance of A26.centre P0
  measures "d8" distance of L31 P0
  measures "d9" distance of P0 L33.end
  measures "d10" distance of L34.start L34.end
extrude "Extrude1" add sketch "Sketch2" along normal blind 2 contours A3 L0 L1 A4 A28 A29 L20 L22 A30 A31 L23 L24 L25 L26 L27 A32 L28 L29 L32 A33 L35 L36 A34 L37 L38 | A28 | A31 | A29 | A30
fillet "Fillet1" radius 3 4 edges at (-20.25, -145.8683, 1) (20.25, -145.8683, 1) (15.7286, -164.6391, 1) (-15.7286, -164.6391, 1)
fillet "Fillet2" radius 2 2 edges at (6, -172.1, 1) (-6, -172.1, 1)
fillet "Fillet3" radius 3 2 edges at (-18.55, -31.7437, 1) (18.55, -31.7437, 1)
fillet "Fillet4" radius 3 2 edges at (-9.756, 4.856, 1) (9.756, 4.856, 1)
fillet "Fillet5" radius 2 1 edges at (0, -4.9, 1)
sketch "Sketch3" plane through (0, 0, 2) normal (0, 0, 1) x (1, 0, 0)
  arc A0 (-7.2751, -171.1221) -> (-4.8986, -171.1648) centre (-6.058, -169.5351) ccw
  arc A1 (4.8986, -171.1648) -> (-4.8986, -171.1648) centre (0, -178.05) ccw
  arc A2 (4.8986, -171.1648) -> (7.2751, -171.1221) centre (6.058, -169.5351) ccw
  line L0 (7.2751, -171.1221) -> (15.0344, -165.1715)
  arc A3 (15.0344, -165.1715) -> (16.0278, -163.817) centre (13.2088, -162.7909) ccw
  line L1 (16.0278, -163.817) -> (19.1143, -155.3371)
  arc A4 (19.1143, -155.3371) -> (19.6835, -152.7386) centre (9.7173, -151.9169) ccw
  line L2 (19.6835, -152.7386) -> (20.2399, -145.9914)
  arc A5 (20.2399, -145.9914) -> (20.25, -145.7449) centre (17.25, -145.7449) ccw
  line L3 (20.25, -145.7449) -> (20.25, -35.5)
  arc A6 (20.25, -35.5) -> (19.1875, -32.4184) centre (15.25, -35.5) ccw
  arc A7 (18.55, -30.5695) -> (19.1875, -32.4184) centre (21.55, -30.5695) ccw
  line L4 (18.55, -30.5695) -> (18.55, 0.8857)
  arc A8 (19, 2.4661) -> (18.55, 0.8857) centre (21.55, 0.8857) ccw
  arc A9 (19, 2.4661) -> (9.7944, 5.7648) centre (14.75, 5.1) ccw
  arc A10 (8.9423, 4.0423) -> (9.7944, 5.7648) centre (6.821, 6.1637) ccw
  line L5 (8.9423, 4.0423) -> (1.4142, -3.4858)
  arc A11 (-1.4142, -3.4858) -> (1.4142, -3.4858) centre (0, -2.0716) ccw
  line L6 (-1.4142, -3.4858) -> (-8.9423, 4.0423)
  arc A12 (-9.7944, 5.7648) -> (-8.9423, 4.0423) centre (-6.821, 6.1637) ccw
  arc A13 (-9.7944, 5.7648) -> (-19, 2.4661) centre (-14.75, 5.1) ccw
  arc A14 (-18.55, 0.8857) -> (-19, 2.4661) centre (-21.55, 0.8857) ccw
  line L7 (-18.55, 0.8857) -> (-18.55, -30.5695)
  arc A15 (-19.1875, -32.4184) -> (-18.55, -30.5695) centre (-21.55, -30.5695) ccw
  arc A16 (-19.1875, -32.4184) -> (-20.25, -35.5) centre (-15.25, -35.5) ccw
  line L8 (-20.25, -35.5) -> (-20.25, -145.7449)
  arc A17 (-20.25, -145.7449) -> (-20.2399, -145.9914) centre (-17.25, -145.7449) ccw
  line L9 (-20.2399, -145.9914) -> (-19.6835, -152.7386)
  arc A18 (-19.6835, -152.7386) -> (-19.1143, -155.3371) centre (-9.7173, -151.9169) ccw
  line L10 (-19.1143, -155.3371) -> (-16.0278, -163.817)
  arc A19 (-16.0278, -163.817) -> (-15.0344, -165.1715) centre (-13.2088, -162.7909) ccw
  line L11 (-15.0344, -165.1715) -> (-7.2751, -171.1221)
  arc A20 (4.253, -18.8853) -> (2.35, -19.8578) centre (3.55, -19.8578) ccw
  line L12 (4.253, -18.8853) -> (8.8217, -22.188)
  arc A21 (9.65, -23.8089) -> (8.8217, -22.188) centre (7.65, -23.8089) ccw
  line L13 (9.65, -23.8089) -> (9.65, -25.2396)
  arc A22 (6.43, -26.8244) -> (9.65, -25.2396) centre (7.65, -25.2396) ccw
  line L14 (6.43, -26.8244) -> (2.818, -24.044)
  arc A23 (2.35, -23.0931) -> (2.818, -24.044) centre (3.55, -23.0931) ccw
  line L15 (2.35, -23.0931) -> (2.35, -19.8578)
  circle A24 centre (11.5, -163.1) radius 1.5
  circle A25 centre (-15.25, -108.3) radius 1.5
  arc A26 (-11.75, -14.5) -> (-9.75, -14.5) centre (-10.75, -14.5) ccw
  line L16 (-11.75, -14.5) -> (-11.75, -2.5)
  arc A27 (-9.75, -2.5) -> (-11.75, -2.5) centre (-10.75, -2.5) ccw
  line L17 (-9.75, -2.5) -> (-9.75, -14.5)
  arc A28 (-13.55, -8.5) -> (-15.55, -8.5) centre (-14.55, -8.5) ccw
  line L18 (-13.55, -8.5) -> (-13.55, -20.5)
  arc A29 (-15.55, -20.5) -> (-13.55, -20.5) centre (-14.55, -20.5) ccw
  line L19 (-15.55, -20.5) -> (-15.55, -8.5)
  circle A30 centre (14.75, 5.1) radius 1.5
  circle A31 centre (15.25, -108.3) radius 1.5
  circle A32 centre (-14.75, 5.1) radius 1.5
  arc A33 (15.55, -8.5) -> (13.55, -8.5) centre (14.55, -8.5) ccw
  line L20 (15.55, -8.5) -> (15.55, -20.5)
  arc A34 (13.55, -20.5) -> (15.55, -20.5) centre (14.55, -20.5) ccw
  line L21 (13.55, -20.5) -> (13.55, -8.5)
  arc A35 (-9.65, -25.2396) -> (-6.43, -26.8244) centre (-7.65, -25.2396) ccw
  line L22 (-9.65, -25.2396) -> (-9.65, -23.8089)
  arc A36 (-8.8217, -22.188) -> (-9.65, -23.8089) centre (-7.65, -23.8089) ccw
  line L23 (-8.8217, -22.188) -> (-4.253, -18.8853)
  arc A37 (-2.35, -19.8578) -> (-4.253, -18.8853) centre (-3.55, -19.8578) ccw
  line L24 (-2.35, -19.8578) -> (-2.35, -23.0931)
  arc A38 (-2.818, -24.044) -> (-2.35, -23.0931) centre (-3.55, -23.0931) ccw
  line L25 (-2.818, -24.044) -> (-6.43, -26.8244)
  circle A39 centre (-15.25, -35.5) radius 1.5
  circle A40 centre (15.25, -35.5) radius 1.5
  circle A41 centre (-11.5, -163.1) radius 1.5
  arc A42 (11.75, -2.5) -> (9.75, -2.5) centre (10.75, -2.5) ccw
  line L26 (11.75, -2.5) -> (11.75, -14.5)
  arc A43 (9.75, -14.5) -> (11.75, -14.5) centre (10.75, -14.5) ccw
  line L27 (9.75, -14.5) -> (9.75, -2.5)